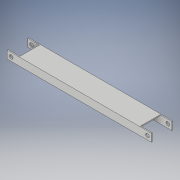
# Autodesk Inventor part: ArmProto2.2Assembly
Saved by Autodesk Inventor 2017 (Build 210142000, 142)
## iProperties
Created: 2017-10-04
Part Number: ArmProto2.2Assembly
Material: Generic
Document SubType Name: Modeling
Designer: User
Density: 1 g/cm^3
Appearance: Default
Author: User
Autodesk Inventor part; units mm, degrees
ref_plane "YZ Plane" through (0, 0, 0) normal (1, 0, 0) x (0, 1, 0)
ref_plane "XZ Plane" through (0, 0, 0) normal (0, 1, 0) x (-1, 0, 0)
ref_plane "XY Plane" through (0, 0, 0) normal (0, 0, 1) x (1, 0, 0)
sketch "Sketch1" plane through (0, 0, 0) normal (1, 0, 0) x (0, 1, 0)
  line L0 (0, 0) -> (25.4, 0)
  line L1 (25.4, 0) -> (25.4, -69.85)
  line L2 (25.4, -69.85) -> (0, -69.85)
  line L3 (0, -69.85) -> (0, 0)
  line L4 (0, -3.175) -> (22.225, -3.175)
  line L5 (22.225, -3.175) -> (22.225, -66.675)
  line L6 (22.225, -66.675) -> (0, -66.675)
  line L7 (0, -66.675) -> (0, -3.175)
  dimension "d0" = 25.4
  dimension "d1" = 69.85
  dimension "d2" = 63.5
  dimension "d3" = 22.225
  dimension "d4" = 3.175
  constraints: 16 end point, 4 parallel, 2 horizontal, 2 perpendicular, 1 point on line
  measures "d0" distance of L1.end L2.end
  measures "d1" distance of L0.end L1.end
  measures "d2" distance of L4.end L5.end
  measures "d3" distance of L5.end L6.end
  measures "d4" distance between parallel lines of L0 L4
extrude "Extrusion1" add sketch "Sketch1" along normal blind 469.9 contours L0 L1 L2 L3 L6 L5 L4
sketch "Sketch3" plane through (0, 25.4, 0) normal (0, 1, 0) x (1, 0, 0)
  line L0 (0, 69.85) -> (0, 0) projected
  line L1 (0, 0) -> (469.9, 0) projected
  line L2 (469.9, 69.85) -> (469.9, 0) projected
  line L3 (0, 69.85) -> (469.9, 69.85) projected
  line L4 (469.9, 3.175) -> (431.8, 3.175)
  line L5 (431.8, 3.175) -> (431.8, 66.675)
  line L6 (431.8, 66.675) -> (469.9, 66.675)
  line L7 (469.9, 66.675) -> (469.9, 3.175)
  line L8 (0, 69.85) -> (0, 0) projected
  line L9 (0, 3.175) -> (38.1, 3.175)
  line L10 (38.1, 3.175) -> (38.1, 66.675)
  line L11 (38.1, 66.675) -> (0, 66.675)
  line L12 (0, 66.675) -> (0, 3.175)
  dimension "d14" = 69.85
  dimension "d16" = 38.1
  dimension "d27" = 38.1
  dimension "d28" = 63.5
  dimension "d29" = 3.175
  dimension "d30" = 63.5
  dimension "d31" = 3.175
  constraints: 16 end point, 4 parallel, 2 horizontal, 2 perpendicular, 2 point on line
  measures "d14" distance of L0.start L0.end
  measures "d16" distance of L5.end L6.end
  measures "d27" distance of L11.end L10.end
  measures "d28" distance of L9.end L10.end
  measures "d29" distance between parallel lines of L3 L11
  measures "d30" distance of L4.end L5.end
  measures "d31" distance between parallel lines of L3 L6
extrude "Extrusion2" cut sketch "Sketch3" against normal blind 3.175 contours L11 L10 L9 L0 | L2 L4 L5 L6
sketch "Sketch4" plane through (0, 0, 0) normal (0, 0, 1) x (1, 0, 0)
  line L0 (0, 25.4) -> (0, 0) projected
  line L1 (0, 0) -> (469.9, 0) projected
  line L2 (469.9, 25.4) -> (469.9, 0) projected
  line L3 (0, 25.4) -> (469.9, 25.4) projected
  circle A0 centre (12.7, 12.7) radius 6.35
  circle A1 centre (457.2, 12.7) radius 6.35
  dimension "d19" = 12.7
  dimension "d20" = 12.7
  dimension "d21" = 25.4
  dimension "d22" = 12.7
  dimension "d23" = 12.7
  dimension "d24" = 12.7
  constraints: 2 centre point
  measures "d19" diameter of A0
  measures "d20" distance from line of L0 A0.centre
  measures "d21" distance of L0.start L0.end
  measures "d22" distance from line of L1 A0.centre
  measures "d23" diameter of A1
  measures "d24" distance from line of L2 A1.centre
extrude "Extrusion3" cut sketch "Sketch4" against normal blind 127 contours A0 | A1
equation "\"d30\" = d28"
equation "\"d31\" = d29"
equation "\"d22\" = 0.5 * d21"
equation "\"d23\" = d20"
equation "\"d24\" = d20"
body "Solid1"
